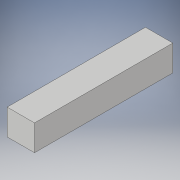
# Autodesk Inventor part: crossbowinsert
Saved by Autodesk Inventor 2018 (Build 220112000, 112)
## iProperties
Created: 2019-03-01
Part Number: crossbowinsert
Material: Generic
Document SubType Name: Modeling
Designer: F8PLTW
Density: 1 g/cm^3
Appearance: Default
Author: F8PLTW
Autodesk Inventor part; units mm, degrees
ref_plane "YZ Plane" through (0, 0, 0) normal (1, 0, 0) x (0, 1, 0)
ref_plane "XZ Plane" through (0, 0, 0) normal (0, 1, 0) x (-1, 0, 0)
ref_plane "XY Plane" through (0, 0, 0) normal (0, 0, 1) x (1, 0, 0)
sketch "Sketch1" plane through (0, 0, 0) normal (0, 0, 1) x (1, 0, 0)
  line L0 (-20.5039, 10.013) -> (-15.9319, 10.013)
  line L1 (-15.9319, 10.013) -> (-15.9319, 5.695)
  line L2 (-15.9319, 5.695) -> (-20.5039, 5.695)
  line L3 (-20.5039, 5.695) -> (-20.5039, 10.013)
  point P0 (0, 0)
  dimension "d0" = 4.572
  dimension "d1" = 4.318
  constraints: 8 end point, 2 parallel, 1 horizontal, 1 perpendicular
  measures "d0" distance of L1.end L2.end
  measures "d1" distance of L0.end L1.end
extrude "Extrusion1" add sketch "Sketch1" along normal blind 23.114
body "Solid1"
